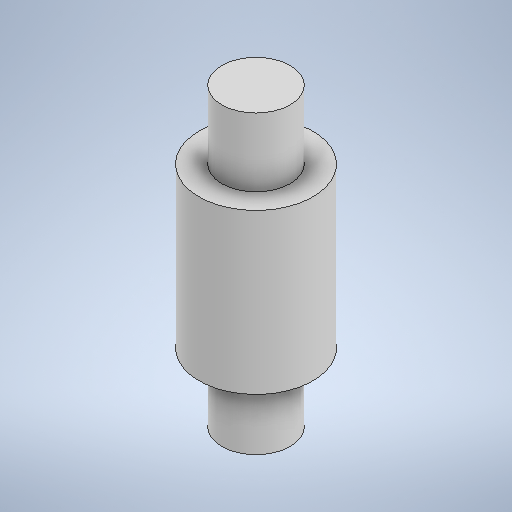
# Autodesk Inventor part: 2063_1
Saved by Autodesk Inventor 2025 (Build 290162010, 162A)
## iProperties
Created: 2024-05-30
Part Number: 2063_1
Material: Generic
Document SubType Name: Modeling
Designer: Fabri
Density: 1 g/cm^3
Appearance: Default
Author: Fabri
Autodesk Inventor part; units mm, degrees
ref_plane "YZ Plane" through (0, 0, 0) normal (1, 0, 0) x (0, 1, 0)
ref_plane "XZ Plane" through (0, 0, 0) normal (0, 1, 0) x (-1, 0, 0)
ref_plane "XY Plane" through (0, 0, 0) normal (0, 0, 1) x (1, 0, 0)
sketch "Sketch1" plane through (0, 0, 0) normal (0, 1, 0) x (-1, 0, 0)
  line L0 (0, 0) -> (1.5, 0)
  line L1 (1.5, 0) -> (1.5, -3)
  line L2 (1.5, -3) -> (2.5, -3)
  line L3 (2.5, -3) -> (2.5, -10)
  line L4 (2.5, -10) -> (1.5, -10)
  line L5 (1.5, -10) -> (1.5, -13)
  line L6 (1.5, -13) -> (0, -13)
  line L7 (0, -13) -> (0, 0)
  point P0 (1.5, -11.5)
  dimension "d1" = 3
  dimension "d2" = 7
  dimension "d3" = 3
  dimension "d4" = 3
  dimension "d5" = 5
  constraints: 16 end point, 5 perpendicular, 2 parallel, 1 horizontal, 1 midpoint, 1 point on line
  measures "d1" distance between parallel lines of L2 L0
  measures "d2" distance of L2.end L3.end
  measures "d3" distance between parallel lines of L4 L6
  measures "d4" diameter of point (1.5, -11.5) L7
  measures "d5" diameter of L3 L7
revolve "Revolution1" add sketch "Sketch1" angle 360 about axis through (0, 0, -13) along (0, 0, 1)
body "Solid1"
